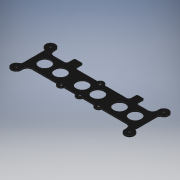
# Autodesk Inventor part: Cover
Saved by Autodesk Inventor 2017 (Build 210142000, 142)
## iProperties
Created: 2017-04-17
Part Number: Cover
Material: Generic
Document SubType Name: Modeling
Designer: jeffkub
Density: 1 g/cm^3
Appearance: Default(1)
Author: jeffkub
Autodesk Inventor part; units mm, degrees
ref_plane "YZ Plane" through (0, 0, 0) normal (1, 0, 0) x (0, 1, 0)
ref_plane "XZ Plane" through (0, 0, 0) normal (0, 1, 0) x (-1, 0, 0)
ref_plane "XY Plane" through (0, 0, 0) normal (0, 0, 1) x (1, 0, 0)
sketch "Sketch1" plane through (0, 0, 0) normal (0, 1, 0) x (-1, 0, 0)
  line L0 (-94, 28.5) -> (94, 28.5) construction
  line L1 (94, 28.5) -> (94, -28.5) construction
  line L2 (94, -28.5) -> (-94, -28.5) construction
  line L3 (-94, -28.5) -> (-94, 17.1863) construction
  line L4 (-94, 28.5) -> (94, -28.5) construction
  line L5 (94, 28.5) -> (-94, -28.5) construction
  arc A0 (86, -28.5) -> (96.6667, -20.9575) centre (94, -28.5) ccw
  arc A1 (96.6667, 20.9575) -> (86, 28.5) centre (94, 28.5) ccw
  arc A2 (-86, 28.5) -> (-96.6667, 20.9575) centre (-94, 28.5) ccw
  arc A3 (-96.6667, -20.9575) -> (-86, -28.5) centre (-94, -28.5) ccw
  line L6 (94, -17.1863) -> (94, 17.1863)
  line L7 (86, -28.5) -> (86, -26)
  line L8 (-86, -26) -> (-86, -28.5)
  line L9 (86, 28.5) -> (86, 26)
  line L10 (-86, 26) -> (-86, 28.5)
  circle A4 centre (13, 0) radius 10
  circle A5 centre (-13, 0) radius 10
  circle A6 centre (49, 0) radius 10
  circle A7 centre (75, 0) radius 10
  circle A8 centre (-49, 0) radius 10
  circle A9 centre (-75, 0) radius 10
  circle A10 centre (0, -16.75) radius 1.9
  circle A11 centre (0, 16.75) radius 1.9
  circle A12 centre (31, 16.75) radius 1.9
  circle A13 centre (-31, 16.75) radius 1.9
  arc A14 (-5.8683, -18) -> (5.8683, -18) centre (0, -16.75) ccw
  arc A15 (5.8683, 18) -> (-5.8683, 18) centre (0, 16.75) ccw
  arc A16 (36.8683, 18) -> (25.1317, 18) centre (31, 16.75) ccw
  arc A17 (-25.1317, 18) -> (-36.8683, 18) centre (-31, 16.75) ccw
  line L11 (78, -18) -> (61, -18)
  line L12 (-5.8683, -18) -> (-42.5, -18)
  line L13 (78, 18) -> (36.8683, 18)
  line L14 (25.1317, 18) -> (5.8683, 18)
  line L15 (-5.8683, 18) -> (-25.1317, 18)
  line L16 (-36.8683, 18) -> (-78, 18)
  arc A18 (86, -26) -> (78, -18) centre (78, -26) ccw
  arc A19 (78, 18) -> (86, 26) centre (78, 26) ccw
  arc A20 (-86, 26) -> (-78, 18) centre (-78, 26) ccw
  arc A21 (-78, -18) -> (-86, -26) centre (-78, -26) ccw
  arc A22 (94, -17.1863) -> (96.6667, -20.9575) centre (98, -17.1863) ccw
  arc A23 (96.6667, 20.9575) -> (94, 17.1863) centre (98, 17.1863) ccw
  arc A24 (-96.6667, -20.9575) -> (-94, -17.1863) centre (-98, -17.1863) ccw
  arc A25 (-94, 17.1863) -> (-96.6667, 20.9575) centre (-98, 17.1863) ccw
  circle A26 centre (94, -28.5) radius 1.6
  circle A27 centre (94, 28.5) radius 1.6
  circle A28 centre (-94, 28.5) radius 1.6
  circle A29 centre (-94, -28.5) radius 1.6
  line L17 (-94, -17.1863) -> (-94, 17.1863)
  line L18 (57, -22) -> (57, -29.5)
  line L19 (55, -31.5) -> (45, -31.5)
  line L20 (43, -29.5) -> (43, -22)
  line L21 (-46.5, -22) -> (-46.5, -29.5)
  line L22 (-48.5, -31.5) -> (-56.5, -31.5)
  line L23 (-58.5, -29.5) -> (-58.5, -22)
  line L24 (39, -18) -> (5.8683, -18)
  line L25 (-62.5, -18) -> (-78, -18)
  arc A30 (55, -31.5) -> (57, -29.5) centre (55, -29.5) ccw
  arc A31 (43, -29.5) -> (45, -31.5) centre (45, -29.5) ccw
  arc A32 (-48.5, -31.5) -> (-46.5, -29.5) centre (-48.5, -29.5) ccw
  arc A33 (-58.5, -29.5) -> (-56.5, -31.5) centre (-56.5, -29.5) ccw
  arc A34 (61, -18) -> (57, -22) centre (61, -22) ccw
  arc A35 (43, -22) -> (39, -18) centre (39, -22) ccw
  arc A36 (-42.5, -18) -> (-46.5, -22) centre (-42.5, -22) ccw
  arc A37 (-58.5, -22) -> (-62.5, -18) centre (-62.5, -22) ccw
  point P0 (0, 0)
  point P1 (94, 20.5)
  point P2 (-94, -20.5)
  point P3 (94, -20.5)
  point P4 (0, 0)
  point P5 (0, 0)
  point P6 (50, -31.5)
  point P7 (-52.5, -31.5)
  point P8 (57, -31.5)
  point P9 (43, -31.5)
  point P10 (43, -18)
  point P11 (-46.5, -31.5)
  point P12 (-58.5, -31.5)
  point P13 (-58.5, -18)
  point P14 (-52.5, -31.5)
  point P15 (50, -31.5)
  dimension "d0" = 188
  dimension "d1" = 57
  dimension "d2" = 20
  dimension "d3" = 26
  dimension "d4" = 13
  dimension "d5" = 36
  dimension "d6" = 26
  dimension "d7" = 36
  dimension "d8" = 26
  dimension "d9" = 8
  dimension "d10" = 16.75
  dimension "d11" = 3.8
  dimension "d12" = 16.75
  dimension "d13" = 31
  dimension "d14" = 31
  dimension "d15" = 12
  dimension "d16" = 18
  dimension "d17" = 18
  dimension "d18" = 8
  dimension "d19" = 4
  dimension "d20" = 3.2
  dimension "d23" = 50
  dimension "d24" = 52.5
  dimension "d25" = 31.5
  dimension "d26" = 14
  dimension "d27" = 12
  dimension "d28" = 2
  dimension "d29" = 4
  constraints: 52 end point, 51 point on circle, 38 centre point, 33 tangent, 29 equal radius, 24 point on line, 14 coincident, 12 perpendicular, 9 horizontal alignment, 7 collinear, 6 midpoint, 6 vertical, 5 horizontal, 3 vertical alignment, 2 parallel
  measures "d0" distance of L1.end L2.end
  measures "d1" distance of L2.end L0.start
  measures "d2" diameter of A5
  measures "d3" distance of A5.centre A4.centre
  measures "d4" distance of point (0, 0) A5.centre
  measures "d5" distance of A8.centre A5.centre
  measures "d6" distance of A9.centre A8.centre
  measures "d7" distance of A6.centre A4.centre
  measures "d8" distance of A7.centre A6.centre
  measures "d9" radius of A0
  measures "d10" distance of A11.centre point (0, 0)
  measures "d11" diameter of A11
  measures "d12" distance of point (0, 0) A10.centre
  measures "d13" distance of A12.centre A11.centre
  measures "d14" distance of A13.centre A11.centre
  measures "d15" diameter of A14
  measures "d16" distance from line of L12 point (0, 0)
  measures "d17" distance from line of L14 point (0, 0)
  measures "d18" radius of A18
  measures "d19" radius of A22
  measures "d20" diameter of A26
  measures "d23" horizontal distance of point (50, -31.5) point (0, 0)
  measures "d24" horizontal distance of point (0, 0) point (-52.5, -31.5)
  measures "d25" vertical distance of point (0, 0) point (-52.5, -31.5)
  measures "d26" distance of point (57, -31.5) point (43, -31.5)
  measures "d27" distance of point (-46.5, -31.5) point (-58.5, -31.5)
  measures "d28" radius of A30
  measures "d29" radius of A34
extrude "Extrusion1" add sketch "Sketch1" along normal blind 1.5
equation "\"d4\" = 0.5 * d3"
equation "\"d6\" = d3"
equation "\"d7\" = d5"
equation "\"d8\" = d3"
equation "\"d12\" = d10"
equation "\"d17\" = d16"
body "Solid1"
